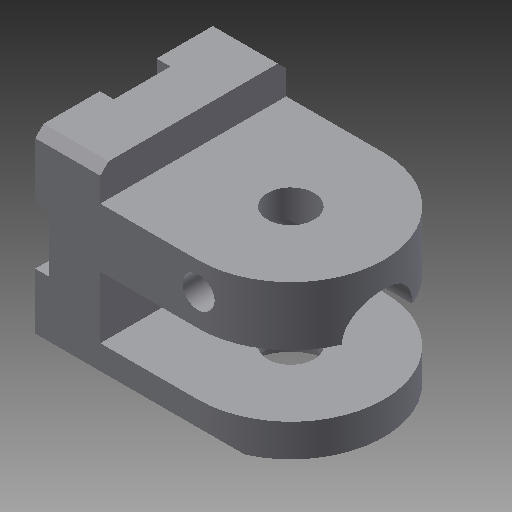
# Autodesk Inventor part: May Tec 1.63.14041_Base plates
Saved by Autodesk Inventor 2018 (Build 220112000, 112)
## iProperties
Category: PARTsolutions
Company: MAYTEC
Created: 2012-12-11
Part Number: May Tec 1.63.14041_Base plates
Catalog Web Link: www.cadenas.de
Description: Joint base corps left-Joint base corps left
Vendor: MAYTEC
Document SubType Name: Modeling
Designer: PARTuser1
Manufacturer: MAYTEC
Density: 1 g/cm^3
Material: Generic
Appearance: RGB(192.00000375509219,192.00000375509219,192.00000375509219)
PSOL_IDENT_0: {\\10.0.0.242\data_v9\23d-libs\maytec\maytec_3d\anbauzubehoer\gelenke\gelenke_pg_30-50_spannhebel\ge
PSOL_IDENT_1: lenk_li_grundkoerper.prj},217 {VTYP=3D},{NB=May Tec 1.63.14041_Base plates},{LINA=May Tec 1.63.14041
PSOL_IDENT_2: _Base plates},{NN=Joint base corps left},{DATE=14.09.2010 08:31:19},{GEOMDATE=15.02.2008 00:00:00},{
PSOL_IDENT_3: VERSION=},{LINEID=60},{LINESUBID=-1},{WBVAR=}  {NB=May Tec 1.63.14041_Base plates},{LINA=May Tec 1.6
PSOL_IDENT_4: 3.14041_Base plates},{KT=DUMMY},{IDNR=},{PARTNR=1.63.14041},{DESCRIPTION=Grundkoerper},{H=40.0},{B=4
PSOL_IDENT_5: 0.0},{L=55.0},{F=1.8},{DS=10.0},{TS=4.0},{DD=8.4},{BN=12.0},{DN=3.0},{SB=11.0},{FI=M8},{FID=6.647},{
PSOL_IDENT_6: D1=15.2},{BL=47.5},{DK=16.8},{A1=7.0},{A2=13.3},{NUT=1.000},{XTRANS=Base plates}
CNS_NT: Joint base corps left
CNS_NB: May Tec 1.63.14041_Base plates
CNS_NBSYN: May Tec $PARTNR._$XTRANS.
CNS_LINA: May Tec 1.63.14041_Base plates
CNS_PARTNR: 1.63.14041
CNS_DESCRIPTION: Base plates
CNS_H: 40.0
CNS_B: 40.0
CNS_L: 55.0
CNS_F: 1.8
CNS_DS: 10.0
CNS_TS: 4.0
CNS_DD: 8.4
CNS_BN: 12.0
CNS_DN: 3.0
CNS_SB: 11.0
CNS_FI: M8
CNS_FID: 6.647
CNS_D1: 15.2
CNS_BL: 47.5
CNS_DK: 16.8
CNS_A1: 7.0
CNS_A2: 13.3
CNS_NUT: 1.000
CNS_XTRANS: Base plates
SUPPLIER: MAYTEC
ARTICLENO: May Tec 1.63.14041_Base plates
BOMINFO: May Tec 1.63.14041_Base plates
CREATOR: CADENAS GmbH
Title: May Tec 1.63.14041_Base plates
Author: Cadenas PARTsolutions
Comments: Joint base corps left
Autodesk Inventor part; units mm, degrees
sketch "Skizze_1" plane through (0, 0, 0) normal (0, 1, 0) x (-1, 0, 0)
  line L0 (35, -20) -> (35, 20)
  line L1 (35, 20) -> (0, 20)
  arc A0 (0, 20) -> (0, -20) centre (0, 0) ccw
  line L2 (0, -20) -> (35, -20)
  constraints: 6 end point, 2 point on circle, 1 centre point
extrude "Extrusion1" add sketch "Skizze_1" along normal mid plane 40
sketch "Skizze_2" plane through (0, 0, 0) normal (0, 0, 1) x (1, 0, 0)
  line L0 (-21, 20) -> (-21, 13)
  line L1 (-21, 13) -> (20, 13)
  line L2 (20, 13) -> (20, 20)
  line L3 (20, 20) -> (-21, 20)
  constraints: 8 end point
extrude "Extrusion2" cut sketch "Skizze_2" along normal mid plane 40
sketch "Skizze_3" plane through (0, 0, 0) normal (0, 0, 1) x (1, 0, 0)
  line L0 (-21, -13) -> (20, -13)
  line L1 (20, -13) -> (20, 0.3)
  line L2 (20, 0.3) -> (-21, 0.3)
  line L3 (-21, 0.3) -> (-21, -13)
  constraints: 8 end point
extrude "Extrusion3" cut sketch "Skizze_3" along normal mid plane 40
sketch "Skizze_4" plane through (20, 0, 0) normal (1, 0, 0) x (0, 0, -1)
  circle A0 centre (0, 0) radius 7.6
  constraints: 1 centre point
extrude "Extrusion4" cut sketch "Skizze_4" against normal blind 47.5
sketch "Sketch5" plane through (-35, -20, -20) normal (-1, 0, 0) x (0, 0, 1)
  point P0 (20, 20)
hole "Drilling 2" at (-35, 0, 0) direction (1, 0, 0) diameter 8.4 depth 11
sketch "Skizze_6" plane through (-35, 0, 0) normal (1, 0, 0) x (0, 0, -1)
  line L0 (-20, -6.1) -> (-6.1, -6.1)
  line L1 (-6.1, -6.1) -> (-6.1, -20)
  line L2 (-6.1, -20) -> (6.1, -20)
  line L3 (6.1, -20) -> (6.1, -6.1)
  line L4 (6.1, -6.1) -> (20, -6.1)
  line L5 (20, -6.1) -> (20, 6.1)
  line L6 (20, 6.1) -> (6.1, 6.1)
  line L7 (6.1, 6.1) -> (6.1, 20)
  line L8 (6.1, 20) -> (-6.1, 20)
  line L9 (-6.1, 20) -> (-6.1, 6.1)
  line L10 (-6.1, 6.1) -> (-20, 6.1)
  line L11 (-20, 6.1) -> (-20, -6.1)
  constraints: 24 end point
extrude "Extrusion5" cut sketch "Skizze_6" along normal blind 3
sketch "Skizze_7" plane through (-35, 0, 0) normal (1, 0, 0) x (0, 0, -1)
  line L0 (18.2, 20) -> (20, 18.2)
  line L1 (20, 18.2) -> (20, 20)
  line L2 (20, 20) -> (18.2, 20)
  constraints: 6 end point
extrude "Extrusion6" cut sketch "Skizze_7" along normal blind 55
sketch "Skizze_8" plane through (-35, 0, 0) normal (1, 0, 0) x (0, 0, -1)
  line L0 (-20, 20) -> (-20, 18.2)
  line L1 (-20, 18.2) -> (-18.2, 20)
  line L2 (-18.2, 20) -> (-20, 20)
  constraints: 6 end point
extrude "Extrusion7" cut sketch "Skizze_8" along normal blind 55
sketch "Skizze_9" plane through (-35, 0, 0) normal (1, 0, 0) x (0, 0, -1)
  line L0 (-20, -20) -> (-18.2, -20)
  line L1 (-18.2, -20) -> (-20, -18.2)
  line L2 (-20, -18.2) -> (-20, -20)
  constraints: 6 end point
extrude "Extrusion8" cut sketch "Skizze_9" along normal blind 55
sketch "Skizze_10" plane through (-35, 0, 0) normal (1, 0, 0) x (0, 0, -1)
  line L0 (18.2, -20) -> (20, -20)
  line L1 (20, -20) -> (20, -18.2)
  line L2 (20, -18.2) -> (18.2, -20)
  constraints: 6 end point
extrude "Extrusion9" cut sketch "Skizze_10" along normal blind 55
sketch "Sketch11" plane through (0, -20, 0) normal (0, -1, 0) x (1, 0, 0)
  point P0 (0, 0)
hole "Drilling 3" at (0, -20, 0) direction (0, 1, 0) diameter 10 depth 40
sketch "Skizze_12" plane through (0, -20, 0) normal (0, 1, 0) x (1, 0, 0)
  circle A0 centre (0, 0) radius 8.4
  constraints: 1 centre point
extrude "Extrusion10" cut sketch "Skizze_12" along normal blind 4
sketch "Skizze_13" plane through (0, 0, 20) normal (0, 0, 1) x (1, 0, 0)
  circle A0 centre (0, 7) radius 3.3235
  constraints: 1 centre point
extrude "Extrusion11" cut sketch "Skizze_13" against normal blind 20
ref_plane "re_XY" through (0, 0, 0) normal (0, 1, 0) x (1, 0, 0)
ref_plane "re_YZ" through (0, 0, 0) normal (1, 0, 0) x (0, 0, -1)
ref_plane "re_ZX" through (0, 0, 0) normal (0, 0, -1) x (0, 1, 0)
ref_plane "bo1_XY" through (0, -20, 0) normal (0, 1, 0) x (1, 0, 0)
ref_plane "bo1_YZ" through (0, -20, 0) normal (1, 0, 0) x (0, 0, -1)
ref_plane "bo1_ZX" through (0, -20, 0) normal (0, 0, -1) x (0, 1, 0)
ref_plane "hebel_XY" through (0, 16, 0) normal (0, 1, 0) x (1, 0, 0)
ref_plane "hebel_YZ" through (0, 16, 0) normal (1, 0, 0) x (0, 0, -1)
ref_plane "hebel_ZX" through (0, 16, 0) normal (0, 0, -1) x (0, 1, 0)
body "Solid1"
